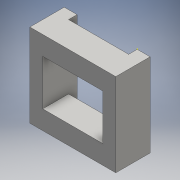
# Autodesk Inventor part: podwozie
Saved by Autodesk Inventor 2016 (Build 200138000, 138)
## iProperties
Created: 2015-11-07
Part Number: podwozie
Material: Ogólny
Document SubType Name: Modeling
Designer: Mrianura
Density: 1 g/cm^3
Appearance: Domyślna
Author: Mrianura
Autodesk Inventor part; units mm, degrees
ref_plane "YZ Plane" through (0, 0, 0) normal (1, 0, 0) x (0, 1, 0)
ref_plane "XZ Plane" through (0, 0, 0) normal (0, 1, 0) x (-1, 0, 0)
ref_plane "XY Plane" through (0, 0, 0) normal (0, 0, 1) x (1, 0, 0)
sketch "Szkic1" plane through (0, 0, 0) normal (0, 1, 0) x (-1, 0, 0)
  line L0 (0, 0) -> (0, -97)
  line L1 (0, -97) -> (70, -97)
  line L2 (70, -97) -> (70, 0)
  line L3 (70, 0) -> (0, 0)
  line L4 (70, 0) -> (85, 0)
  line L5 (85, 0) -> (85, -97)
  line L6 (85, -97) -> (70, -97)
  line L7 (0, -97) -> (-15, -97)
  line L8 (-15, -97) -> (-15, 0)
  line L9 (-15, 0) -> (0, 0)
  line L10 (70, 0) -> (70, -25)
  line L11 (70, -25) -> (0, -25)
  line L12 (70, -97) -> (70, -72)
  line L13 (70, -72) -> (0, -72)
  line L14 (70, -48.5) -> (70, -72.5)
  line L15 (70, -48.5) -> (70, -24.5)
  line L16 (0, -48.5) -> (0, -72.5)
  line L17 (0, -48.5) -> (0, -24.5)
  dimension "d0" = 97
  dimension "d1" = 70
  dimension "d2" = 15
  dimension "d3" = 15
  dimension "d4" = 25
  dimension "d5" = 25
  dimension "d6" = 24
  dimension "d7" = 24
  dimension "d8" = 24
  dimension "d9" = 24
  constraints: 36 end point, 12 point on line, 9 perpendicular, 2 midpoint, 1 vertical
  measures "d0" distance of L0.start L0.end
  measures "d1" distance of L0.end L1.end
  measures "d2" distance of L2.end L4.end
  measures "d3" distance of L0.end L7.end
  measures "d4" distance of L2.end L10.end
  measures "d5" distance of L1.end L12.end
  measures "d6" distance of L14.start L14.end
  measures "d7" distance of L14.start L15.end
  measures "d8" distance of L16.start L16.end
  measures "d9" distance of L16.start L17.end
extrude "Wyciągnięcie proste1" add sketch "Szkic1" along normal blind 40 contours L0 L7 L8 L9 | L4 L5 L6 L2
sketch "Szkic2" plane through (0, 40, 0) normal (0, 1, 0) x (1, 0, 0)
  point P0 (0, 0)
sketch "Szkic3" plane through (0, 0, 0) normal (0, -1, 0) x (1, 0, 0)
  line L0 (-70, 0) -> (-70, -97) projected
  line L1 (-70, 0) -> (-70, -22)
  line L2 (-70, -22) -> (0, -22)
  line L3 (0, -97) -> (0, 0) projected
  line L4 (0, -22) -> (0, 0)
  line L5 (0, 0) -> (-70, 0)
  line L6 (-70, -97) -> (-70, -75)
  line L7 (-70, -75) -> (0, -75)
  line L8 (0, -97) -> (-70, -97)
  dimension "d12" = 22
  dimension "d13" = 22
  constraints: 14 end point, 3 perpendicular, 3 point on line, 1 collinear, 1 parallel
  measures "d12" distance of L0.start L1.end
  measures "d13" distance of L0.end L6.end
extrude "Wyciągnięcie proste2" add sketch "Szkic3" against normal blind 30 contours L5 L3 L2 L0 | L7 L3 L8 L0
